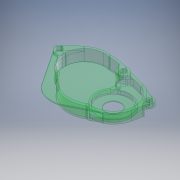
# Autodesk Inventor part: body gauche
Saved by Autodesk Inventor 2018.1 (Build 221171000, 171)
## iProperties
Created: 2022-07-20
Part Number: body gauche
Material: Generic
Document SubType Name: Modeling
Designer: mouta
Density: 1 g/cm^3
Appearance: Default
Mass: 46.6039 g
Surface Area: 416.174 cm^2
Volume: 46.6039 cm^3
Author: mouta
Autodesk Inventor part; units mm, degrees
ref_plane "YZ Plane" through (0, 0, 0) normal (1, 0, 0) x (0, 1, 0)
ref_plane "XZ Plane" through (0, 0, 0) normal (0, 1, 0) x (-1, 0, 0)
ref_plane "XY Plane" through (0, 0, 0) normal (0, 0, 1) x (1, 0, 0)
sketch "Sketch1" plane through (0, 0, 0) normal (0, 0, 1) x (1, 0, 0)
  circle A0 centre (0, 0) radius 5
  circle A1 centre (149.4, 0) radius 5
  circle A2 centre (85.7991, 21.6971) radius 5
  circle A3 centre (110.2989, -19.8991) radius 12.5
  arc A4 (154.885, -2.4321) -> (154.9491, -2.282) centre (149.4, 0) ccw
  line L0 (-1.9594, 5.6711) -> (-0.9713, 5.9209)
  line L1 (94.051, 25.713) -> (120.8026, 18.6971)
  arc A5 (131.5219, 14.0064) -> (120.0887, 18.8843) centre (110.2989, -19.8991) ccw
  line L2 (0, 0) -> (4.8474, 1.2258)
  line L3 (80.8741, 20.8344) -> (85.7991, 21.6971)
  arc A6 (125.9738, -56.7) -> (149.4311, -28.1861) centre (110.2989, -19.8991) ccw
  line L4 (80.7723, -79.2884) -> (129.3991, -55.0443)
  line L5 (-2.1405, -7.4309) -> (37.9799, -67.1663)
  arc A7 (90.3858, 23.6876) -> (86.8225, 21.8764) centre (110.2989, -19.8991) ccw
  arc A8 (33.9775, -61.2072) -> (80.7723, -79.2884) centre (68.0362, -42.6558) ccw
  arc A9 (-3.2331, 6.2086) -> (-3.6699, -5.9609) centre (0, 0) ccw
  line L6 (131.5219, 14.0064) -> (145.3135, 8.2114)
  line L7 (150.7621, 5.922) -> (151.3594, 5.6711)
  line L8 (154.928, -2.2287) -> (154.885, -2.4321)
  line L9 (153.6652, -8.1921) -> (149.4311, -28.1861)
  arc A10 (154.9491, -2.282) -> (154.3356, -0.8001) centre (110.2989, -19.8991) ccw
  arc A11 (151.6581, 4.4611) -> (150.7621, 5.922) centre (110.2989, -19.8991) ccw
  arc A12 (-0.9713, 5.9209) -> (-1.9594, 5.6711) centre (0, 0) ccw
  arc A13 (-4.6746, 3.7614) -> (-4.9033, 3.458) centre (55.8634, -42.1071) ccw
  arc A14 (-4.6746, 3.7614) -> (-4.9033, 3.458) centre (0, 0) ccw
  arc A15 (-3.2331, 6.2086) -> (-1.7498, 7.3852) centre (-5.5425, 10.6433) ccw
  arc A16 (-2.1405, -7.4309) -> (-3.6699, -5.9609) centre (-6.2912, -10.2187) ccw
  arc A17 (50.3563, 33.7779) -> (18.6552, 24.2587) centre (44.1835, -3.2106) ccw
  arc A18 (80.9569, 29.5804) -> (51.4686, 33.7181) centre (55.8634, -42.1071) ccw
  arc A19 (17.7599, 23.5959) -> (-1.7498, 7.3852) centre (55.8634, -42.1071) ccw
  arc A20 (17.7599, 23.5959) -> (18.6552, 24.2587) centre (15.2515, 27.9212) ccw
  arc A21 (50.3563, 33.7779) -> (51.4686, 33.7181) centre (51.1793, 38.7097) ccw
  arc A22 (91.6578, 27.1447) -> (83.8358, 29.4525) centre (85.7991, 21.6971) ccw
  arc A23 (155.0349, -5.6787) -> (148.0771, 7.8899) centre (149.4, 0) ccw
  arc A24 (155.0349, -5.6787) -> (153.6652, -8.1921) centre (158.5567, -9.2279) ccw
  arc A25 (145.3135, 8.2114) -> (148.0771, 7.8899) centre (147.2503, 12.821) ccw
  arc A26 (80.9569, 29.5804) -> (83.8358, 29.4525) centre (82.6088, 34.2996) ccw
  arc A27 (91.6578, 27.1447) -> (94.051, 25.713) centre (95.3194, 30.5494) ccw
  point P0 (90.8386, 26.5555)
  point P1 (111.3369, -59.8857)
  point P2 (-4.37, -4.1113)
  point P3 (148.3758, 6.9247)
  point P4 (154.3524, -4.9471)
  point P5 (-2.8318, -6.4017)
  point P6 (92.4582, 26.1307)
  point P7 (146.8277, 7.5752)
  point P8 (154.0164, -6.5337)
  dimension "d3" = 10
  dimension "d5" = 10
  dimension "d15" = 10
  dimension "d18" = 25
  dimension "d20" = 12
  dimension "d88" = 14
  dimension "d104" = 75
  dimension "d105" = 5
  dimension "d112" = 16
  dimension "d113" = 16
  dimension "d114" = 5
  constraints: 61 point on circle, 27 centre point, 20 end point, 17 tangent, 10 point on line, 6 coincident, 4 equal radius, 3 other
  measures "d5" diameter of A1
  measures "d15" diameter of A2
  measures "d18" diameter of A3
  measures "d20" diameter of A4
  measures "d88" diameter of A9
  measures "d104" diameter of A17
  measures "d105" radius of A20
  measures "d112" diameter of A22
  measures "d113" diameter of A23
  measures "d114" radius of A24
extrude "Extrusion2" add sketch "Sketch1" along normal blind 21 contours L8 A10 A4 | L1 A5 L6 A25 A23 A24 L9 A6 L4 A8 L5 A16 A9 A15 A19 A20 A17 A21 A18 A26 A22 A27 | A13 A14
sketch "Sketch13" plane through (0, 0, 21) normal (0, 0, 1) x (1, 0, 0)
  arc A0 (105.7808, -55.6145) -> (122.4659, 13.9825) centre (110.2989, -19.8991) ccw
  line L0 (32.2727, -40.0871) -> (32.3131, -38.891)
  circle A1 centre (85.7991, 21.6971) radius 5 projected
  arc A2 (122.3009, 14.0385) -> (99.574, 19.2733) centre (79.666, -119.1093) ccw
  arc A3 (75.8354, 22.6759) -> (71.8549, 28.0781) centre (70.8606, 23.1779) ccw
  arc A4 (99.574, 19.2733) -> (94.503, 16.7734) centre (98.8621, 14.3243) ccw
  arc A5 (105.7808, -55.6145) -> (100.6423, -58.4183) centre (105.1533, -60.575) ccw
  arc A6 (32.3131, -38.891) -> (31.6808, -35.0382) centre (22.3188, -38.553) ccw
  arc A7 (71.8549, 28.0781) -> (53.5859, 30.1834) centre (55.1609, -36.4655) ccw
  arc A8 (45.4593, 29.5658) -> (46.2806, 29.608) centre (45.6146, 34.5634) ccw
  arc A9 (122.4659, 13.9825) -> (122.3009, 14.0385) centre (120.7761, 9.2767) ccw
  arc A10 (32.2727, -40.0871) -> (100.6423, -58.4183) centre (68.36, -42.1569) ccw
  arc A11 (75.8354, 22.6759) -> (94.503, 16.7734) centre (85.7848, 21.6718) ccw
  arc A12 (21.1272, 20.7085) -> (21.4488, 20.9624) centre (18.1914, 24.7558) ccw
  arc A13 (26.215, -29.3432) -> (26.5512, -29.4928) centre (38.2081, -2.8397) ccw
  arc A14 (52.3785, 30.3021) -> (53.5859, 30.1834) centre (53.4677, 35.182) ccw
  arc A15 (31.6808, -35.0382) -> (28.8407, -32.1468) centre (26.9998, -36.7956) ccw
  arc A16 (10.959, -0.9486) -> (11, 0) centre (0, 0) ccw
  arc A17 (42.9394, 31.1577) -> (11, 0) centre (44.2313, -2.1157) ccw
  arc A18 (11, 0) -> (28.1802, -31.8274) centre (45.4352, -1.9627) ccw
  arc A19 (52.3785, 30.3021) -> (42.9394, 31.1577) centre (44.3663, -5.5943) ccw
  arc A20 (28.1802, -31.8274) -> (28.8407, -32.1468) centre (30.6816, -27.498) ccw
  point P0 (44.2138, -2.45)
  point P1 (68.1634, -42.8903)
  point P2 (32.5739, -31.1818)
  dimension "d97" = 5
  dimension "d99" = 10
  dimension "d106" = 5
  dimension "d107" = 5
  dimension "d108" = 5
  dimension "d111" = 5
  dimension "d149" = 22
  dimension "d150" = 5
  constraints: 42 point on circle, 20 centre point, 12 tangent, 3 equal radius, 2 coincident, 2 end point, 1 point on line
  measures "d97" radius of A3
  measures "d99" radius of A6
  measures "d106" radius of A8
  measures "d107" radius of A9
  measures "d108" radius of A12
  measures "d111" radius of A14
  measures "d149" diameter of A16
  measures "d150" radius of A20
extrude "Extrusion18" cut sketch "Sketch13" against normal blind 30 contours A5 A10 L0 A6 A15 A20 A18 A16 A17 A19 A14 A7 A3 A11 A4 A2 A9 A0
sketch "Sketch14" plane through (0, 0, 0) normal (0, 0, -1) x (-1, 0, 0)
  arc A0 (-149.4311, -28.1861) -> (-129.3991, -55.0443) centre (-110.2989, -19.8991) ccw projected
  arc A1 (-119.4387, 14.9213) -> (-106.6539, -55.7141) centre (-110.2989, -19.8991) ccw
  arc A2 (-106.2146, -55.6889) -> (-106.6539, -55.7141) centre (-106.1477, -60.6885) ccw
  arc A3 (-40.8348, -42.3354) -> (-40.8163, -42.4047) centre (-32.2727, -40.0871) ccw
  arc A4 (-32.4708, -39.2737) -> (-32.4771, -39.299) centre (-30.9909, -39.6595) ccw
  arc A5 (-99.574, 19.2733) -> (-122.3009, 14.0385) centre (-79.666, -119.1093) ccw projected
  arc A6 (-99.574, 19.2733) -> (-122.3009, 14.0385) centre (-79.666, -119.1093) ccw
  arc A7 (-94.503, 16.7734) -> (-99.574, 19.2733) centre (-98.8621, 14.3243) ccw projected
  arc A8 (-94.503, 16.7734) -> (-99.574, 19.2733) centre (-98.8621, 14.3243) ccw
  arc A9 (-94.503, 16.7734) -> (-75.8354, 22.6759) centre (-85.7848, 21.6718) ccw projected
  arc A10 (-94.503, 16.7734) -> (-94.503, 16.7734) centre (-85.7848, 21.6718) ccw
  arc A11 (-71.8549, 28.0781) -> (-75.8354, 22.6759) centre (-70.8606, 23.1779) ccw projected
  arc A12 (-71.8549, 28.0781) -> (-75.8354, 22.6759) centre (-70.8606, 23.1779) ccw
  arc A13 (-53.5859, 30.1834) -> (-71.8549, 28.0781) centre (-55.1609, -36.4655) ccw
  arc A14 (-42.9394, 31.1577) -> (-52.3785, 30.3021) centre (-44.3663, -5.5943) ccw projected
  arc A15 (-7.6133, -6.0028) -> (-7.5869, -5.4513) centre (-12.5868, -5.4886) ccw projected
  arc A16 (-7.6133, -6.0028) -> (-7.5869, -5.4513) centre (-12.5868, -5.4886) ccw
  arc A17 (-53.5859, 30.1834) -> (-52.3785, 30.3021) centre (-53.4677, 35.182) ccw projected
  arc A18 (-52.3785, 30.3021) -> (-52.3785, 30.3021) centre (-53.4677, 35.182) ccw
  arc A19 (-122.4659, 13.9825) -> (-105.7808, -55.6145) centre (-110.2989, -19.8991) ccw projected
  arc A20 (-104.4615, -55.6231) -> (-105.7808, -55.6145) centre (-105.1533, -60.575) ccw
  line L0 (-102.236, -56.6732) -> (-99.574, -66.0535)
  line L1 (-99.574, -66.0535) -> (-89.7348, -73.9688)
  line L2 (-89.7348, -73.9688) -> (-70.8599, -80.5455)
  line L3 (-70.8599, -80.5455) -> (-50.5074, -76.4133)
  line L4 (-50.5074, -76.4133) -> (-38.2081, -66.0535)
  line L5 (-38.2081, -66.0535) -> (-31.6808, -53.4239)
  arc A21 (-29.3298, -32.1761) -> (-40.7919, -42.2064) centre (-26.4301, -47.054) ccw
  arc A22 (-101.9177, -56.7625) -> (-40.9149, -42.4525) centre (-79.2709, -16.1237) ccw
  line L6 (-102.2342, -56.6549) -> (-102.1958, -56.5806)
  arc A23 (-100.6423, -58.4183) -> (-105.7808, -55.6145) centre (-105.1533, -60.575) ccw projected
  line L7 (-102.1581, -56.5725) -> (-101.921, -56.7603)
  arc A24 (-102.2342, -56.6549) -> (-102.236, -56.6732) centre (-102.212, -56.6664) ccw
  arc A25 (-102.1581, -56.5725) -> (-102.1958, -56.5806) centre (-102.1736, -56.5921) ccw
  arc A26 (-101.921, -56.7603) -> (-101.9177, -56.7625) centre (-101.9055, -56.7407) ccw
  arc A27 (-27.7299, -31.5655) -> (-22.9163, -28.0988) centre (-45.091, -2.3837) ccw
  arc A28 (-29.3298, -32.1761) -> (-27.7299, -31.5655) centre (-30.2864, -27.2685) ccw
  line L8 (-31.6808, -53.4239) -> (-21.3438, -29.2493)
  arc A29 (-28.1802, -31.8274) -> (-10.959, -0.9486) centre (-45.4352, -1.9627) ccw projected
  arc A30 (-21.3438, -29.2493) -> (-22.9163, -28.0988) centre (-22.2632, -28.8562) ccw
  arc A31 (-40.9149, -42.4525) -> (-40.7919, -42.2064) centre (-41.7393, -41.8866) ccw
  point P0 (0, 0)
  point P1 (-68.36, -42.1569)
  point P2 (-44.3656, -5.7255)
  point P3 (-32.331, -38.4801)
  point P4 (-102.2925, -56.4742)
  point P5 (-102.2925, -56.4742)
  point P6 (-102.2387, -56.6637)
  point P7 (-102.1818, -56.5537)
  point P8 (-101.9194, -56.7615)
  point P9 (-19.3004, -24.4706)
  dimension "d117" = 5
  dimension "d151" = 0.025
  dimension "d152" = 5
  dimension "d153" = 1
  dimension "d154" = 1
  constraints: 47 point on circle, 19 centre point, 18 end point, 13 tangent, 7 point on line, 2 coincident, 2 equal radius, 10 other
  measures "d117" radius of A2
  measures "d151" radius of A24
  measures "d152" radius of A28
  measures "d153" radius of A30
  measures "d154" radius of A31
extrude "Extrusion19" add sketch "Sketch14" against normal blind 21 contours A24 L6 A25 A23 A22 A31 A21 A28 A27 A30 L8 L5 L4 L3 L2 L1 L0
sketch "Sketch15" plane through (0, 0, 0) normal (0, 0, -1) x (-1, 0, 0)
  arc A0 (-102.1107, -56.5406) -> (-102.1047, -56.5437) centre (-102.0961, -56.5203) ccw
  arc A1 (-34.3648, -42.1416) -> (-34.3673, -42.1438) centre (-34.3499, -42.1617) ccw
  arc A2 (-105.7089, -55.6248) -> (-105.7097, -55.6249) centre (-105.7065, -55.6497) ccw
  arc A3 (-128.0312, -55.6155) -> (-105.8763, -57.6335) centre (-113.5213, -18.9414) ccw
  line L0 (-18.6552, 24.2587) -> (18.4437, 24.2587)
  line L1 (18.4437, -18.7212) -> (18.4437, -89.3277)
  line L2 (17.4437, -90.3277) -> (-128.3991, -90.3277)
  line L3 (-129.3991, -89.3277) -> (-129.3991, -56.5453)
  arc A4 (-103.1642, -58.2909) -> (-39.2846, -43.6103) centre (-79.2093, -16.2059) ccw
  arc A5 (-28.7087, -34.0675) -> (-39.2002, -43.4615) centre (-23.1542, -50.8264) ccw
  arc A6 (-28.5801, -34.0146) -> (-11.105, -14.574) centre (-44.2263, -2.3758) ccw
  arc A7 (-28.7087, -34.0675) -> (-28.5801, -34.0146) centre (-29.0233, -33.1182) ccw
  arc A8 (-39.2846, -43.6103) -> (-39.2002, -43.4615) centre (-40.1091, -43.0444) ccw
  arc A9 (-128.0312, -55.6155) -> (-129.3991, -56.5453) centre (-128.3991, -56.5453) ccw
  arc A10 (-105.7205, -57.6153) -> (-105.8763, -57.6335) centre (-105.6825, -58.6145) ccw
  arc A11 (-129.3991, -89.3277) -> (-128.3991, -90.3277) centre (-128.3991, -89.3277) ccw
  arc A12 (17.4437, -90.3277) -> (18.4437, -89.3277) centre (17.4437, -89.3277) ccw
  arc A13 (-103.2814, -58.2128) -> (-105.611, -57.605) centre (-105.1584, -60.6391) ccw
  arc A14 (-105.7205, -57.6153) -> (-105.611, -57.605) centre (-105.7586, -56.616) ccw
  arc A15 (-103.2814, -58.2128) -> (-103.1642, -58.2909) centre (-102.6695, -57.4218) ccw
  line L4 (0.1556, -6.7212) -> (6.4437, -6.7212)
  arc A16 (0.1556, -6.7212) -> (-11.105, -14.574) centre (0.1556, -18.7212) ccw
  arc A17 (18.4437, -18.7212) -> (6.4437, -6.7212) centre (6.4437, -18.7212) ccw
  point P0 (0, 0)
  point P1 (-32.4771, -39.299)
  point P2 (-17.7599, 23.5959)
  point P3 (-7.5869, -5.4513)
  point P4 (-129.3991, -55.0443)
  point P5 (-10.959, -0.9486)
  dimension "d159" = 1
  dimension "d160" = 1
  dimension "d162" = 1
  dimension "d163" = 1
  dimension "d164" = 1
  dimension "d165" = 12
  constraints: 37 point on circle, 19 tangent, 18 centre point, 10 end point, 5 equal radius, 3 perpendicular, 2 horizontal, 1 point on line
  measures "d159" radius of A7
  measures "d160" radius of A8
  measures "d162" radius of A9
  measures "d163" radius of A11
  measures "d164" radius of A14
  measures "d165" radius of A16
extrude "Extrusion21" cut sketch "Sketch15" against normal blind 19 contours A3 A10 A14 A13 A15 A4 A8 A5 A7 A6 A16 L4 A17 L1 A12 L2 A11 L3 A9
sketch "Sketch17" plane through (0, 0, 0) normal (0, 0, -1) x (-1, 0, 0)
  line L0 (-118.5538, 17.4586) -> (-97.5506, 20.785)
  line L1 (-97.5506, 20.785) -> (-92.4179, 17.4222)
  line L2 (-92.4179, 17.4222) -> (-89.5328, 13.7993)
  line L3 (-89.5328, 13.7993) -> (-83.6174, 13.1723)
  line L4 (-83.6174, 13.1723) -> (-79.5039, 16.4479)
  line L5 (-79.5039, 16.4479) -> (-77.3189, 19.783)
  line L6 (-77.3189, 19.783) -> (-78.0733, 24.5465)
  line L7 (-78.0733, 24.5465) -> (-75.8354, 27.9624)
  line L8 (-75.8354, 27.9624) -> (-68.4126, 30.6179)
  line L9 (-68.4126, 30.6179) -> (-53.5502, 31.8272)
  line L10 (-53.5502, 31.8272) -> (-44.0663, 32.5989)
  line L11 (-44.0663, 32.5989) -> (-33.4554, 30.9363)
  line L12 (-33.4554, 30.9363) -> (-20.8096, 24.5465)
  line L13 (-20.8096, 24.5465) -> (-10.2105, 7.6353)
  line L14 (-10.2105, 7.6353) -> (-10.2105, -5.5162)
  line L15 (-10.2105, -5.5162) -> (-11.4311, -13.3062)
  line L16 (-11.4311, -13.3062) -> (-16.1982, -22.7406)
  line L17 (-16.1982, -22.7406) -> (-24.4891, -30.7296)
  line L18 (-24.4891, -30.7296) -> (-32.1287, -34.2561)
  line L19 (-32.1287, -34.2561) -> (-38.6971, -40.5854)
  line L20 (-38.6971, -40.5854) -> (-43.3312, -46.4515)
  line L21 (-43.3312, -46.4515) -> (-52.3837, -55.1744)
  line L22 (-52.3837, -55.1744) -> (-64.0767, -61.0812)
  line L23 (-64.0767, -61.0812) -> (-79.0974, -63.9302)
  line L24 (-79.0974, -63.9302) -> (-92.0242, -61.9047)
  line L25 (-92.0242, -61.9047) -> (-98.0201, -59.7947)
  line L26 (-98.0201, -59.7947) -> (-103.3966, -57.078)
  line L27 (-103.3966, -57.078) -> (-104.2007, -56.6717)
  line L28 (-104.2007, -56.6717) -> (-108.1669, -56.9944)
  line L29 (-108.1669, -56.9944) -> (-117.7995, -56.6717)
  line L30 (-117.7995, -56.6717) -> (-127.157, -53.9466)
  line L31 (-127.157, -53.9466) -> (-137.7031, -45.2155)
  line L32 (-137.7031, -45.2155) -> (-144.0104, -36.5561)
  line L33 (-144.0104, -36.5561) -> (-147.8732, -21.2399)
  line L34 (-147.8732, -21.2399) -> (-149.8502, -10.8162)
  line L35 (-149.8502, -10.8162) -> (-145.9418, -6.0953)
  line L36 (-145.9418, -6.0953) -> (-142.9558, -1.5377)
  line L37 (-142.9558, -1.5377) -> (-139.9648, 6.9616)
  line L38 (-139.9648, 6.9616) -> (-132.9824, 10.9671)
  line L39 (-132.9824, 10.9671) -> (-126.2428, 14.3717)
  line L40 (-126.2428, 14.3717) -> (-118.998, 17.3344)
  arc A0 (-118.5538, 17.4586) -> (-118.998, 17.3344) centre (-118.241, 15.4832) ccw
  point P0 (0, 0)
  dimension "d168" = 2
  constraints: 82 end point, 9 perpendicular, 6 parallel, 5 point on line, 2 point on circle, 2 tangent, 1 centre point, 1 vertical
  measures "d168" radius of A0
extrude "Extrusion22" add sketch "Sketch17" against normal blind 1.4
sketch "Sketch18" plane through (0, 0, 1.4) normal (0, 0, 1) x (1, 0, 0)
  arc A0 (105.7808, -55.6145) -> (122.4659, 13.9825) centre (110.2989, -19.8991) ccw projected
  arc A1 (107.702, -55.8054) -> (120.9774, 14.4807) centre (110.2989, -19.8991) ccw
  circle A2 centre (110.2989, -19.8991) radius 26
  arc A3 (100.7929, 19.893) -> (97.8909, 20.7198) centre (96.6936, 11.0118) ccw
  arc A4 (119.2402, 15.4307) -> (103.7963, 19.5158) centre (107.1931, 1.1219) ccw
  arc A5 (100.7929, 19.893) -> (103.7963, 19.5158) centre (102.8883, 24.4327) ccw
  arc A6 (119.2402, 15.4307) -> (120.9774, 14.4807) centre (122.4605, 19.2556) ccw
  arc A7 (87.8059, -1.5944) -> (94.3476, -44.118) centre (110.2989, -19.8991) ccw
  line L0 (94.3476, -44.118) -> (104.5174, -54.3442)
  line L1 (87.2237, 7.5392) -> (87.8059, -1.5944)
  arc A8 (104.5174, -54.3442) -> (107.702, -55.8054) centre (108.0627, -50.8184) ccw
  circle A9 centre (85.7991, 21.6971) radius 5 projected
  arc A10 (87.2237, 7.5392) -> (83.4295, 12.076) centre (82.2338, 7.2211) ccw
  line L2 (83.4295, 12.076) -> (94.3891, 19.8378)
  arc A11 (97.8909, 20.7198) -> (94.3891, 19.8378) centre (97.2789, 15.7574) ccw
  point P0 (0, 0)
  point P1 (86.9485, 11.8554)
  point P2 (105.7808, -55.6145)
  point P3 (95.6613, 20.7388)
  dimension "d171" = 52
  dimension "d194" = 58
  dimension "d195" = 5
  dimension "d197" = 5
  dimension "d198" = 5
  constraints: 22 point on circle, 10 centre point, 9 tangent, 6 end point, 3 coincident, 3 point on line, 1 equal radius
  measures "d171" diameter of A2
  measures "d194" diameter of A7
  measures "d195" radius of A8
  measures "d197" radius of A10
  measures "d198" radius of A11
extrude "Extrusion24" add sketch "Sketch18" along normal blind 7 contours A8 L0 A7 L1 A10 L2 A11 A3 A5 A4 A6 A1 A0
sketch "Sketch19" plane through (110.2989, -19.8991, 1.4) normal (0, 0, 1) x (1, 0, 0)
  circle A0 centre (0, 0) radius 13
  point P0 (-110.2989, 19.8991)
  dimension "d177" = 26
  constraints: 1 centre point
  measures "d177" diameter of A0
extrude "Extrusion25" cut sketch "Sketch19" against normal blind 2
sketch "Sketch20" plane through (0, 0, 0) normal (0, 0, -1) x (-1, 0, 0)
  circle A0 centre (-149.4, 0) radius 5 projected
  circle A1 centre (-85.7991, 21.6971) radius 5 projected
  circle A2 centre (0, 0) radius 10
  arc A3 (-148.0771, 7.8899) -> (-145.3135, 8.2114) centre (-147.2503, 12.821) ccw projected
  arc A4 (-93.7288, 17.4405) -> (-76.9386, 23.2758) centre (-85.7991, 21.6971) ccw
  arc A5 (-76.7762, 25.6832) -> (-95.3493, 19.2282) centre (-88.4937, 29.4504) ccw
  arc A6 (-93.7288, 17.4405) -> (-95.3493, 19.2282) centre (-98.1343, 15.0757) ccw
  arc A7 (-76.7762, 25.6832) -> (-76.9386, 23.2758) centre (-72.0161, 24.1528) ccw
  line L0 (-149.4311, -28.1861) -> (-153.6652, -8.1921) projected
  line L1 (-145.3135, 8.2114) -> (-131.5219, 14.0064) projected
  arc A8 (-151.8902, -10.5463) -> (-141.6974, 8.3767) centre (-155.5075, 3.6088) ccw
  arc A9 (-141.8947, 10.8793) -> (-154.0886, -11.7585) centre (-182.2622, 18.0201) ccw
  arc A10 (-141.8947, 10.8793) -> (-141.6974, 8.3767) centre (-136.9712, 10.0084) ccw
  arc A11 (-151.8902, -10.5463) -> (-154.0886, -11.7585) centre (-150.6523, -15.3906) ccw
  dimension "d182" = 20
  dimension "d188" = 18
  dimension "d189" = 5
  dimension "d190" = 5
  constraints: 16 point on circle, 9 centre point, 8 tangent, 2 coincident, 2 equal radius
  measures "d182" diameter of A2
  measures "d188" diameter of A4
  measures "d189" radius of A6
  measures "d190" radius of A10
extrude "Extrusion28" cut sketch "Sketch20" against normal blind 14
sketch "Sketch22" plane through (0, 0, 0) normal (0, 0, -1) x (-1, 0, 0)
  line L0 (-98.5192, 37.356) -> (-143.6597, 16.7031)
  line L1 (-145.5287, 15.2228) -> (-165.0948, -9.9765)
  line L2 (-165.9493, -14.4301) -> (-155.5318, -50.5048)
  line L3 (-151.7096, -54.0203) -> (-125.2843, -59.3107)
  line L4 (-87.4011, 30.5456) -> (-88.8223, 13.0293)
  line L5 (-88.8223, 13.0293) -> (-89.0582, 9.6195)
  arc A0 (-96.4364, 5.573) -> (-121.0722, -46.8238) centre (-110.2989, -19.8991) ccw
  arc A1 (-96.4364, 5.573) -> (-89.0582, 9.6195) centre (-94.0463, 9.9647) ccw
  line L6 (-90.3003, 35.4947) -> (-94.3545, 37.3541)
  arc A2 (-87.4011, 30.5456) -> (-90.3003, 35.4947) centre (-92.3848, 30.9499) ccw
  arc A3 (-94.3545, 37.3541) -> (-98.5192, 37.356) centre (-96.4389, 32.8093) ccw
  arc A4 (-143.6597, 16.7031) -> (-145.5287, 15.2228) centre (-141.5794, 12.1564) ccw
  arc A5 (-165.0948, -9.9765) -> (-165.9493, -14.4301) centre (-161.1455, -13.0429) ccw
  arc A6 (-155.5318, -50.5048) -> (-151.7096, -54.0203) centre (-150.728, -49.1176) ccw
  arc A7 (-118.5913, -48.9803) -> (-111.4546, -55.9735) centre (-102.6416, -39.8417) ccw
  line L7 (-116.3488, -64.402) -> (-123.6637, -59.9439)
  arc A8 (-109.2559, -62.3307) -> (-111.4546, -55.9735) centre (-113.8517, -60.3615) ccw
  arc A9 (-116.3488, -64.402) -> (-109.2559, -62.3307) centre (-113.7467, -60.1325) ccw
  arc A10 (-118.5913, -48.9803) -> (-121.0722, -46.8238) centre (-122.9296, -51.466) ccw
  arc A11 (-123.6637, -59.9439) -> (-125.2843, -59.3107) centre (-126.2659, -64.2134) ccw
  point P0 (0, 0)
  point P1 (-92.3812, 2.9034)
  point P2 (-110.2989, -48.8991)
  point P3 (-89.6892, 0.5027)
  point P4 (-103.2814, -58.2128)
  point P5 (-107.1169, -57.6708)
  dimension "d201" = 5
  dimension "d202" = 5
  dimension "d203" = 5
  dimension "d204" = 5
  dimension "d205" = 5
  constraints: 27 point on circle, 17 tangent, 16 end point, 12 centre point, 5 equal radius, 1 coincident, 1 point on line
  measures "d201" radius of A1
  measures "d202" radius of A2
  measures "d203" radius of A8
  measures "d204" radius of A10
  measures "d205" radius of A11
extrude "Extrusion29" cut sketch "Sketch22" against normal blind 5
sketch "Sketch23" plane through (0, 0, 0) normal (0, 0, -1) x (-1, 0, 0)
  arc A0 (-28.5801, -34.0146) -> (-11.105, -14.574) centre (-44.2263, -2.3758) ccw projected
  arc A1 (-18.6552, 24.2587) -> (-17.7599, 23.5959) centre (-15.2515, 27.9212) ccw projected
  arc A2 (-11.105, -14.574) -> (-18.6552, 24.2587) centre (-51.4476, -2.2675) ccw
  line L0 (-18.6552, 24.2587) -> (-22.3178, 27.6624)
  arc A3 (-18.6552, 24.2587) -> (-50.3563, 33.7779) centre (-44.1835, -3.2106) ccw projected
  line L1 (-22.3178, 27.6624) -> (-15.1248, 27.6624)
  line L2 (-15.1248, 27.6624) -> (11.504, 9.7162)
  line L3 (11.504, 9.7162) -> (11.504, -7.4142)
  line L4 (11.504, -7.4142) -> (4.7165, -25.9717)
  line L5 (4.7165, -25.9717) -> (-11.105, -14.574)
  point P0 (0, 0)
  dimension "d208" = 5
  constraints: 12 end point, 2 point on circle, 1 centre point, 1 horizontal, 1 perpendicular, 1 tangent
  measures "d208" distance of L0.start L0.end
extrude "Extrusion30" cut sketch "Sketch23" against normal blind 14
body "Solid2"
